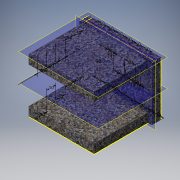
# Autodesk Inventor part: BaseMini
Saved by Autodesk Inventor 2016 (Build 200138000, 138)
## iProperties
Created: 2015-08-01
Part Number: BaseMini
Material: Concrete
Document SubType Name: Modeling
Designer: myhome
Density: 2.40731 g/cm^3
Appearance: Exposed Aggregate - Coarse
Mass: 40442.8 g
Surface Area: 8020 cm^2
Volume: 16800 cm^3
Author: myhome
Autodesk Inventor part; units mm, degrees
ref_plane "YZ Plane" through (0, 0, 0) normal (1, 0, 0) x (0, 1, 0)
ref_plane "XZ Plane" through (0, 0, 0) normal (0, 1, 0) x (-1, 0, 0)
ref_plane "XY Plane" through (0, 0, 0) normal (0, 0, 1) x (1, 0, 0)
sketch "Sketch1" plane through (0, 0, 0) normal (0, 0, 1) x (1, 0, 0)
  line L0 (0, 0) -> (400, 0)
  line L1 (400, 0) -> (400, 300)
  line L2 (400, 300) -> (0, 300)
  line L3 (0, 300) -> (0, 0)
  line L4 (400, 150) -> (0, 150) construction
  line L5 (200, 300) -> (200, 0) construction
  dimension "d0" = 400
  dimension "d1" = 300
  constraints: 12 end point, 4 midpoint, 2 parallel, 1 horizontal, 1 perpendicular
  measures "d0" distance of L1.end L2.end
  measures "d1" distance of L0.end L1.end
extrude "Extrusion1" add sketch "Sketch1" along normal blind 50
sketch "Sketch2" plane through (0, 0, 0) normal (0, 1, 0) x (-1, 0, 0)
  line L0 (0, 50) -> (-400, 50) projected
  line L1 (0, 50) -> (-20, 50)
  line L2 (-20, 50) -> (-20, 350)
  line L3 (-20, 350) -> (-380, 350)
  line L4 (-380, 350) -> (-380, 50)
  point P0 (0, 0)
  dimension "d4" = 20
  dimension "d5" = 300
  dimension "d6" = 360
  constraints: 8 end point, 3 perpendicular, 2 point on line
  measures "d4" distance of L0.start L1.end
  measures "d5" distance of L1.end L2.end
  measures "d6" distance of L2.end L3.end
sketch "Sketch3" plane through (0, 0, 0) normal (0, 1, 0) x (-1, 0, 0)
  line L0 (-20, 50) -> (-20, 350) projected
  line L1 (-20, 350) -> (-380, 350) projected
  line L2 (-380, 350) -> (-380, 50) projected
  point P0 (0, 0)
extrude "Extrusion2" add sketch "Sketch2" along normal blind 50
ref_plane "Work Plane1" through (0, 150, 0) normal (0, -1, 0) x (1, 0, 0)
ref_plane "Work Plane2" through (0, 300, 0) normal (0, -1, 0) x (1, 0, 0)
sketch "Sketch4" plane through (0, 300, 0) normal (0, -1, 0) x (1, 0, 0)
  line L0 (20, 350) -> (380, 350) projected
  line L1 (380, 350) -> (380, 50) projected
  line L2 (20, 50) -> (20, 350) projected
  line L3 (380, 50) -> (20, 50)
  line L4 (400, 50) -> (0, 50) projected
  point P0 (0, 0)
  constraints: 2 end point, 1 collinear
extrude "Extrusion3" add sketch "Sketch4" along normal blind 50
sketch "Sketch5" plane through (0, 300, 0) normal (0, 1, 0) x (1, 0, 0)
  line L0 (400, 0) -> (400, -50) projected
  line L1 (400, 0) -> (400, -25)
  line L2 (400, -25) -> (350, -25)
  line L3 (350, -25) -> (300, -25)
  line L4 (300, -25) -> (250, -25)
  line L5 (250, -25) -> (200, -25)
  line L6 (200, -25) -> (150, -25)
  line L7 (150, -25) -> (100, -25)
  line L8 (100, -25) -> (50, -25)
  line L9 (50, -25) -> (0, -25)
  line L10 (0, 0) -> (0, -50) projected
  dimension "d12" = 50
  dimension "d13" = 50
  dimension "d14" = 50
  dimension "d15" = 50
  dimension "d16" = 50
  dimension "d17" = 50
  dimension "d18" = 50
  constraints: 18 end point, 6 point on line, 2 midpoint, 1 horizontal
  measures "d12" distance of L1.end L2.end
  measures "d13" distance of L2.end L3.end
  measures "d14" distance of L3.end L4.end
  measures "d15" distance of L4.end L5.end
  measures "d16" distance of L5.end L6.end
  measures "d17" distance of L6.end L7.end
  measures "d18" distance of L7.end L8.end
sketch "Sketch6" plane through (0, 0, 0) normal (0, -1, 0) x (1, 0, 0)
  line L0 (0, 0) -> (0, 25)
  line L1 (0, 0) -> (0, 50) projected
  line L2 (0, 25) -> (50, 25)
  line L3 (50, 25) -> (100, 25)
  line L4 (100, 25) -> (150, 25)
  line L5 (150, 25) -> (200, 25)
  line L6 (200, 25) -> (250, 25)
  line L7 (250, 25) -> (300, 25)
  line L8 (300, 25) -> (350, 25)
  line L9 (350, 25) -> (400, 25)
  dimension "d19" = 50
  dimension "d20" = 50
  dimension "d21" = 50
  dimension "d22" = 50
  dimension "d23" = 50
  dimension "d24" = 50
  dimension "d25" = 50
  dimension "d26" = 50
  constraints: 18 end point, 7 point on line, 1 horizontal, 1 midpoint
  measures "d19" distance of L0.end L2.end
  measures "d20" distance of L2.end L3.end
  measures "d21" distance of L3.end L4.end
  measures "d22" distance of L4.end L5.end
  measures "d23" distance of L5.end L6.end
  measures "d24" distance of L6.end L7.end
  measures "d25" distance of L7.end L8.end
  measures "d26" distance of L8.end L9.end
sketch "Sketch8" plane through (20, 0, 50) normal (-1, 0, 0) x (0, 0, 1)
  line L0 (0, 0) -> (0, 50) projected
  line L1 (0, 25) -> (50, 25)
  line L2 (50, 25) -> (100, 25)
  line L3 (100, 25) -> (150, 25)
  line L4 (150, 25) -> (200, 25)
  line L5 (200, 25) -> (250, 25)
  point P0 (-50, 0)
  dimension "d27" = 50
  dimension "d28" = 50
  dimension "d29" = 50
  dimension "d30" = 50
  dimension "d31" = 50
  constraints: 10 end point, 3 horizontal, 2 point on line, 1 midpoint
  measures "d27" distance of L1.start L1.end
  measures "d28" distance of L1.end L2.end
  measures "d29" distance of L2.end L3.end
  measures "d30" distance of L3.end L4.end
  measures "d31" distance of L4.end L5.end
sketch "Sketch9" plane through (20, 300, 50) normal (-1, 0, 0) x (0, 0, 1)
  line L0 (-50, 0) -> (0, 0) projected
  line L1 (0, 0) -> (0, -25)
  line L2 (0, 0) -> (0, -300) projected
  line L3 (0, -25) -> (50, -25)
  line L4 (50, -25) -> (100, -25)
  line L5 (100, -25) -> (150, -25)
  line L6 (150, -25) -> (200, -25)
  line L7 (200, -25) -> (250, -25)
  point P0 (-50, -300)
  dimension "d32" = 25
  dimension "d33" = 50
  dimension "d34" = 50
  dimension "d35" = 50
  dimension "d36" = 50
  dimension "d37" = 50
  constraints: 12 end point, 5 point on line, 1 perpendicular
  measures "d32" distance of L0.end L1.end
  measures "d33" distance of L1.end L3.end
  measures "d34" distance of L3.end L4.end
  measures "d35" distance of L4.end L5.end
  measures "d36" distance of L5.end L6.end
  measures "d37" distance of L6.end L7.end
sketch "Sketch11" plane through (0, 0, 0) normal (0, 0, 1) x (1, 0, 0)
  line L0 (400, 0) -> (400, 300) projected
  circle A0 centre (200, 150) radius 25 construction
  line L1 (200, 150) -> (140, 150) construction
  line L2 (140, 150) -> (130, 150) construction
  line L3 (130, 150) -> (110, 150) construction
  line L4 (200, 150) -> (260, 150) construction
  line L5 (260, 150) -> (270, 150)
  line L6 (270, 150) -> (290, 150) construction
  point P0 (0, 0)
  dimension "d38" = 50
  dimension "d39" = 60
  dimension "d40" = 10
  dimension "d41" = 20
  dimension "d42" = 60
  dimension "d43" = 10
  dimension "d44" = 20
  constraints: 12 end point, 4 point on line, 2 horizontal, 1 centre point
  measures "d38" diameter of A0
  measures "d39" distance of L1.start L1.end
  measures "d40" distance of L1.end L2.end
  measures "d41" distance of L2.end L3.end
  measures "d42" distance of L1.start L4.end
  measures "d43" distance of L4.end L5.end
  measures "d44" distance of L5.end L6.end
ref_plane "Work Plane3" through (0, 0, 50) normal (0, 0, -1) x (-1, 0, 0)
sketch "Sketch13" plane through (0, 0, 50) normal (0, 0, -1) x (-1, 0, 0)
  circle A0 centre (-200, 150) radius 25 construction
  line L0 (-200, 150) -> (-140, 150) construction
  line L1 (-140, 150) -> (-130, 150) construction
  line L2 (-130, 150) -> (-110, 150) construction
  line L3 (-200, 150) -> (-260, 150) construction
  line L4 (-260, 150) -> (-270, 150) construction
  line L5 (-270, 150) -> (-290, 150) construction
  line L6 (-290, 150) -> (-300, 150)
  line L7 (-110, 150) -> (-100, 150)
  point P0 (0, 0)
  dimension "d46" = 10
  dimension "d47" = 10
  constraints: 4 end point, 2 horizontal
  measures "d46" distance of L5.end L6.end
  measures "d47" distance of L2.end L7.end
body "Solid1"
